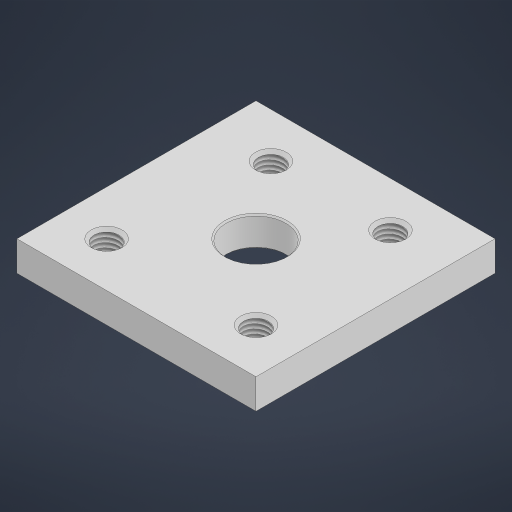
# Autodesk Inventor part: AP1-001
Saved by Autodesk Inventor 2024.3 (Build 283343000, 343)
## iProperties
Created: 2024-05-02
Part Number: AP1-001
Material: Generic
Document SubType Name: Modeling
Designer: fablabadmin
Density: 1 g/cm^3
Appearance: Default
Description: Plate bottom
Author: fablabadmin
Autodesk Inventor part; units mm, degrees
ref_plane "YZ Plane" through (0, 0, 0) normal (1, 0, 0) x (0, 1, 0)
ref_plane "XZ Plane" through (0, 0, 0) normal (0, 1, 0) x (-1, 0, 0)
ref_plane "XY Plane" through (0, 0, 0) normal (0, 0, 1) x (1, 0, 0)
sketch "Sketch1" plane through (0, 0, 0) normal (0, 1, 0) x (-1, 0, 0)
  line L0 (-40, 40) -> (40, 40)
  line L1 (40, 40) -> (40, -40)
  line L2 (40, -40) -> (-40, -40)
  line L3 (-40, -40) -> (-40, 40)
  line L4 (-40, 40) -> (40, -40) construction
  line L5 (40, 40) -> (-40, -40) construction
  line L6 (-25, 25) -> (25, 25) construction
  line L7 (25, 25) -> (25, -25) construction
  line L8 (25, -25) -> (-25, -25) construction
  line L9 (-25, -25) -> (-25, 25) construction
  line L10 (-25, 25) -> (25, -25) construction
  line L11 (25, 25) -> (-25, -25) construction
  circle A0 centre (0, 0) radius 10
  line L12 (20, 25) -> (-20, 25)
  line L13 (-20, 25) -> (-20, -25) construction
  line L14 (-20, -25) -> (20, -25) construction
  line L15 (20, -25) -> (20, 25) construction
  line L16 (56, 0) -> (-56, 0) construction
  line L17 (0, -56) -> (0, 56) construction
  dimension "d0" = 80
  dimension "d1" = 50
  dimension "d2" = 20
  dimension "d12" = 40
  constraints: 32 end point, 6 parallel, 5 coincident, 4 midpoint, 4 perpendicular, 3 horizontal, 3 point on line, 1 centre point, 1 other
  measures "d0" distance of L1.end L2.end
  measures "d1" distance of L7.end L8.end
  measures "d2" diameter of A0
  measures "d12" distance between parallel lines of L15 L13
extrude "Extrusion1" add sketch "Sketch1" against normal blind 10
hole "Hole1" at (-25, 0, 25) at (25, 0, 25) at (-20, 0, -25) at (20, 0, -25) direction (0, -1, 0) diameter 8.376 end through all thread size "M10x1.5" class "6H" standard "ISO Metric profile"
chamfer "Chamfer1" distance 1 angle 45 8 edges at (-20, 0, -29.188) (20, 0, -29.188) (25, 0, 20.812) (-25, 0, 20.812) (-25, -10, 20.812) (-20, -10, -29.188) (20, -10, -29.188) (25, -10, 20.812)
chamfer "Chamfer2" distance 0.5 angle 45 2 edges at (10, 0, 0) (10, -10, 0)
body "Solid1"
